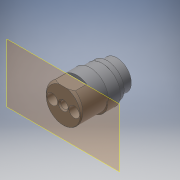
# Autodesk Inventor part: cycloid_input_cam_onepart
Saved by Autodesk Inventor 2019.4 (Build 234330000, 330)
## iProperties
Created: 2019-08-28
Part Number: cycloid_input_cam_onepart
Material: Generic
Document SubType Name: Modeling
Designer: cdi
Density: 1 g/cm^3
Appearance: Default
Author: cdi
Autodesk Inventor part; units mm, degrees
ref_plane "YZ Plane" through (0, 0, 0) normal (1, 0, 0) x (0, 1, 0)
ref_plane "XZ Plane" through (0, 0, 0) normal (0, 1, 0) x (-1, 0, 0)
sketch "Sketch1" plane through (0, 0, 0) normal (0, 0, 1) x (1, 0, 0)
  circle A0 centre (0, 0) radius 1.5
  line L0 (0, 0) -> (0, 0.5)
  circle A1 centre (0, 0.5) radius 7.495
  dimension "d0" = 3
  dimension "d1" = 0.5
  dimension "d2" = 14.99
  constraints: 2 centre point, 2 coincident, 2 end point, 1 vertical
  measures "d0" diameter of A0
  measures "d1" distance of L0.start L0.end
  measures "d2" diameter of A1
extrude "Extrusion1" add sketch "Sketch1" along normal blind 14
sketch "Sketch2" plane through (0, 0, 0) normal (1, 0, 0) x (0, 1, 0)
  line L0 (-6.995, 0) -> (-6.995, 14) projected
  line L1 (-6.995, 11) -> (-10.995, 11)
  line L2 (-10.995, 11) -> (-10.995, 7)
  line L3 (-10.995, 7) -> (-6.995, 7)
  line L4 (-6.995, 7) -> (-6.995, 11)
  line L5 (-6.995, 11) -> (-10.995, 7)
  line L6 (0, -2.8) -> (0, 16.8) projected
  line L7 (-6.995, 0) -> (-6.995, 14) projected
  line L8 (-6.995, 11) -> (-10.995, 11)
  line L9 (-10.995, 11) -> (-10.995, 14)
  line L10 (-10.995, 14) -> (-6.995, 14)
  line L11 (-6.995, 14) -> (-6.995, 11)
  point P0 (0, 0)
  dimension "d5" = 3
  dimension "d6" = 4
  dimension "d7" = 4
  dimension "d58" = 0
  constraints: 18 end point, 4 parallel, 2 horizontal, 2 perpendicular, 2 point on line
  measures "d5" distance from line of L0.end L1
  measures "d6" distance of L1.start L1.end
  measures "d7" distance of L1.end L2.end
  measures "d58" distance from line of L7.end L10
revolve "Revolution1" cut sketch "Sketch2" angle 360 about axis through (0, 0, -10) along (0, 0, 1) contours L1 L9 L10 L0 | L5 L2 L1
sketch "Sketch3" plane through (0, 0.5, 0) normal (0, 0, -1) x (-1, 0, 0)
  line L0 (0, -0.5) -> (0, -1)
  circle A0 centre (0, -1) radius 7.495
  circle A1 centre (0, -0.5) radius 1.5 projected
  circle A2 centre (0, 0) radius 7.495 projected
  dimension "d10" = 14.99
  dimension "d13" = 0.5
  constraints: 2 end point, 1 centre point, 1 coincident, 1 vertical
  measures "d10" diameter of A0
  measures "d13" distance of L0.start L0.end
extrude "Extrusion2" add sketch "Sketch3" along normal blind 5 contours A0 A2 | A2 A0 picked at (-0.4539, -8.1042) picked at (5.3809, 0.0672)
chamfer "Chamfer1" distance 0.5 angle 45 1 edges at (0, -6.995, 0)
sketch "Sketch7" plane through (0, -0.5, -5) normal (0, 0, -1) x (-1, 0, 0)
  circle A0 centre (0, 0.5) radius 6.995
  circle A1 centre (0, 0.5) radius 1.5 projected
  circle A2 centre (0, 0) radius 7.495 projected
  dimension "d120" = 0.5
  constraints: 1 centre point, 1 coincident, 1 tangent
  measures "d120" distance of point (0, 0.5) A2.centre
extrude "Extrusion6" add sketch "Sketch7" along normal blind 2 contours A0
sketch "Sketch8" plane through (0, 0, -7) normal (0, 0, -1) x (-1, 0, 0)
  circle A0 centre (0, 0) radius 1.5 projected
  circle A1 centre (0, 0) radius 5.96
  dimension "d36" = 11.92
  constraints: 1 centre point, 1 coincident
  measures "d36" diameter of A1
extrude "Extrusion7" add sketch "Sketch8" along normal blind 4
sketch "Sketch9" plane through (0, 0, 14) normal (0, 0, 1) x (1, 0, 0)
  line L0 (17, 4) -> (-17, 4)
  line L1 (-17, 4) -> (-17, -4)
  line L2 (-17, -4) -> (17, -4)
  line L3 (17, -4) -> (17, 4)
  line L4 (17, 4) -> (-17, -4) construction
  line L5 (-17, 4) -> (17, -4) construction
  circle A0 centre (17, 0) radius 4
  circle A1 centre (-17, 0) radius 4
  circle A2 centre (0, 0) radius 1.5 projected
  dimension "d39" = 34
  dimension "d40" = 8
  constraints: 12 end point, 4 midpoint, 2 parallel, 2 vertical alignment, 1 horizontal, 1 perpendicular, 4 other
  measures "d39" distance of L2.end L1.end
  measures "d40" distance of L1.end L0.end
extrude "Extrusion8" add sketch "Sketch9" along normal blind 2
sketch "Sketch10" plane through (0, 0, 16) normal (0, 0, 1) x (1, 0, 0)
  line L0 (17, 4) -> (-17, 4) projected
  arc A0 (-17, 4) -> (-17, -4) centre (-17, 0) ccw projected
  line L1 (-17, -4) -> (17, -4) projected
  arc A1 (17, -4) -> (17, 4) centre (17, 0) ccw projected
  circle A2 centre (17, 0) radius 4
  circle A3 centre (-17, 0) radius 4
  point P0 (0, 0)
  dimension "d43" = 8
  dimension "d44" = 8
  constraints: 2 centre point, 2 coincident
  measures "d43" diameter of A2
  measures "d44" diameter of A3
extrude "Extrusion9" add sketch "Sketch10" along normal blind 1.5 contours A1 A2 | A3 A0
sketch "Sketch11" plane through (0, 0, 14) normal (0, 0, -1) x (-1, 0, 0)
  circle A0 centre (-17, 0) radius 4 projected
  circle A1 centre (17, 0) radius 4 projected
  point P0 (0, 0)
hole "Hole1" at (17, 0, 14) at (-17, 0, 14) direction (0, 0, 1) diameter 3.1 depth 10 countersink diameter 6.5 countersink angle 90
sketch "Sketch12" plane through (0, 0, 16) normal (0, 0, 1) x (1, 0, 0)
  circle A0 centre (0, 0) radius 10
  circle A1 centre (0, 0) radius 1.5 projected
  dimension "d59" = 20
  constraints: 1 centre point, 1 coincident
  measures "d59" diameter of A0
extrude "Extrusion10" add sketch "Sketch12" against normal up to surface (2 mm away)
sketch "Sketch13" plane through (0, 0, 16) normal (0, 0, 1) x (1, 0, 0)
  line L0 (-12, 7.5) -> (12, 7.5)
  line L1 (12, 7.5) -> (12, -7.5)
  line L2 (12, -7.5) -> (-12, -7.5)
  line L3 (-12, -7.5) -> (-12, 7.5)
  line L4 (-12, 7.5) -> (12, -7.5) construction
  line L5 (12, 7.5) -> (-12, -7.5) construction
  point P0 (0, 0)
  dimension "d63" = 24
  dimension "d64" = 15
  constraints: 12 end point, 2 midpoint, 2 parallel, 1 horizontal, 1 perpendicular
  measures "d63" distance of L1.end L2.end
  measures "d64" distance of L0.end L1.end
extrude "Extrusion11" add sketch "Sketch13" against normal up to surface (2 mm away)
fillet "Fillet7" radius 2 1 edges at (0, 6.995, 14)
sketch "Sketch16" plane through (0, 0, 16) normal (0, 0, 1) x (1, 0, 0)
  arc A0 (17, 4) -> (17, -4) centre (17, 0) ccw projected
  line L0 (-12, 4) -> (-17, 4) projected
  line L1 (-17, -4) -> (-12, -4) projected
  line L2 (-12, -7.5) -> (-12, -4) projected
  line L3 (-6.6144, -7.5) -> (-12, -7.5) projected
  arc A1 (-6.6144, -7.5) -> (6.6144, -7.5) centre (0, 0) ccw projected
  line L4 (12, -7.5) -> (6.6144, -7.5) projected
  line L5 (12, -4) -> (12, -7.5) projected
  line L6 (12, -4) -> (17, -4) projected
  line L7 (17, 4) -> (12, 4) projected
  line L8 (12, 7.5) -> (12, 4) projected
  line L9 (6.6144, 7.5) -> (12, 7.5) projected
  arc A2 (6.6144, 7.5) -> (-6.6144, 7.5) centre (0, 0) ccw projected
  line L10 (-12, 7.5) -> (-6.6144, 7.5) projected
  line L11 (-12, 4) -> (-12, 7.5) projected
  arc A3 (-17, -4) -> (-17, 4) centre (-17, 0) ccw projected
  line L12 (-12, -7.5) -> (-12, -4) projected
  line L13 (-12, -4) -> (-12, 4)
  line L14 (12, -4) -> (12, 4)
  constraints: 4 end point, 1 collinear, 1 parallel
extrude "Extrusion13" add sketch "Sketch16" along normal blind 3 contours L14 L5 L4 A1 L3 L2 L13 L11 L10 A2 L9 L8
sketch "Sketch17" plane through (0, 0, 19) normal (0, 0, 1) x (1, 0, 0)
  line L0 (12, 7.5) -> (12, 4) projected
  line L1 (-12, -5.05) -> (12, -5.05)
  line L2 (12, -5.05) -> (12, 5.05)
  line L3 (12, 5.05) -> (-12, 5.05)
  line L4 (-12, 5.05) -> (-12, -5.05)
  line L5 (-12, -5.05) -> (12, 5.05) construction
  line L6 (12, -5.05) -> (-12, 5.05) construction
  point P0 (0, 0)
  dimension "d76" = 10.1
  constraints: 12 end point, 2 midpoint, 2 parallel, 1 horizontal, 1 perpendicular, 1 point on line
  measures "d76" distance of L2.end L1.end
extrude "Extrusion14" cut sketch "Sketch17" against normal up to surface (3 mm away)
fillet "Fillet9" radius 2 16 edges at (12, 7.5, 17.5) (12, 7.5, 15) (-6.6144, 7.5, 17.5) (-6.6144, 7.5, 15) (6.6144, 7.5, 17.5) (6.6144, 7.5, 15) (-12, 7.5, 17.5) (-12, 7.5, 15) (12, -7.5, 15) (12, -7.5, 17.5) (-6.6144, -7.5, 15) (-6.6144, -7.5, 17.5) (6.6144, -7.5, 15) (6.6144, -7.5, 17.5) (-12, -7.5, 15) (-12, -7.5, 17.5)
sketch "Sketch18" plane through (0, 0, -11) normal (0, 0, -1) x (-1, 0, 0)
  circle A0 centre (0, 0) radius 4.5
  circle A1 centre (0, 0) radius 1.5 projected
  dimension "d80" = 9
  constraints: 1 centre point, 1 coincident
  measures "d80" diameter of A0
extrude "Extrusion15" add sketch "Sketch18" along normal blind 5.5
sketch "Sketch19" plane through (0, 0, -16.5) normal (0, 0, -1) x (-1, 0, 0)
  circle A0 centre (0, 0) radius 3.05
  dimension "d83" = 6.1
  constraints: 1 centre point, 1 coincident
  measures "d83" diameter of A0
extrude "Extrusion16" cut sketch "Sketch19" against normal blind 3
sketch "Sketch20" plane through (0, 0, -13.5) normal (0, 0, -1) x (-1, 0, 0)
  circle A0 centre (0, 0) radius 1.5 projected
extrude "Extrusion17" cut sketch "Sketch20" against normal through all
fillet "Fillet10" radius 1 6 edges at (14.5, -4, 14) (14.5, 4, 14) (21, 0, 14) (-21, 0, 14) (-14.5, -4, 14) (-14.5, 4, 14)
fillet "Fillet11" radius 1 8 edges at (12, -3.7071, 14.2929) (12, -4, 15.5) (12, 3.7071, 14.2929) (12, 4, 15.5) (-12, 3.7071, 14.2929) (-12, 4, 15.5) (-12, -3.7071, 14.2929) (-12, -4, 15.5)
ref_plane "Work Plane1" through (0, 0, 11) normal (0, 0, 1) x (1, 0, 0)
sketch "Sketch21" plane through (0, 0, 11) normal (0, 0, 1) x (1, 0, 0)
  line L0 (25.9282, -18.0093) -> (-26.8099, -18.0093)
  line L1 (-26.8099, -18.0093) -> (-26.8099, 22.6464)
  line L2 (-26.8099, 22.6464) -> (25.9282, 22.6464)
  line L3 (25.9282, 22.6464) -> (25.9282, -18.0093)
  point P0 (0, 0)
  constraints: 8 end point, 2 parallel, 1 horizontal, 1 perpendicular
extrude "Extrusion18" cut sketch "Sketch21" along normal through all
sketch "Sketch22" plane through (0, 0, 11) normal (0, 0, 1) x (1, 0, 0)
  circle A0 centre (0, 0) radius 1.5 projected
  circle A1 centre (0, 0) radius 1.55
  dimension "d93" = 3.1
  constraints: 1 centre point, 1 coincident
  measures "d93" diameter of A1
extrude "Extrusion19" cut sketch "Sketch22" against normal through all
sketch "Sketch23" plane through (0, 0, 11) normal (0, 0, 1) x (1, 0, 0)
  circle A0 centre (-4.5, 0) radius 1.5
  point P0 (0, 0)
  dimension "d96" = 3
  dimension "d97" = 4.5
  constraints: 1 centre point
  measures "d96" diameter of A0
  measures "d97" distance of point (0, 0) A0.centre
hole "Hole2" at (-4.5, 0, 11) direction (0, 0, -1) diameter 3.88 depth 7 countersink diameter 4.34 countersink angle 7
pattern_circular "Circular Pattern1" count 2 over 360 about axis through (0, 0, 11) along (0, 0, -1) of "Hole2"
chamfer "Chamfer4" distance 0.5 angle 45 1 edges at (-1.55, 0, 11)
sketch "Sketch24" plane through (0, 0, -16.5) normal (0, 0, -1) x (-1, 0, 0)
  circle A0 centre (0, 0) radius 17.4266
  constraints: 1 centre point, 1 coincident
extrude "Extrusion20" cut sketch "Sketch24" against normal up to surface (5.5 mm away)
sketch "Sketch27" plane through (0, 0, 11) normal (0, 0, 1) x (1, 0, 0)
  line L0 (8.8228, 0) -> (-11.4628, 0)
  line L1 (10.8975, 6.8) -> (-11.7772, 6.8)
  line L2 (6.8551, 6.8) -> (-10.3114, 6.8)
  line L3 (-10.3114, 6.8) -> (-10.3114, 10.1454)
  line L4 (-10.3114, 10.1454) -> (6.8551, 10.1454)
  line L5 (6.8551, 10.1454) -> (6.8551, 6.8)
  point P0 (0, 0)
  dimension "d121" = 6.8
  constraints: 12 end point, 3 horizontal, 3 parallel, 1 perpendicular, 1 point on line
  measures "d121" distance between parallel lines of L0 L1
extrude "Extrusion24" cut sketch "Sketch27" against normal blind 5.6
equation "\"d1\" = E_"
equation "\"d13\" = E_"
equation "\"E_\" = 0.5"
body "Solid1"
